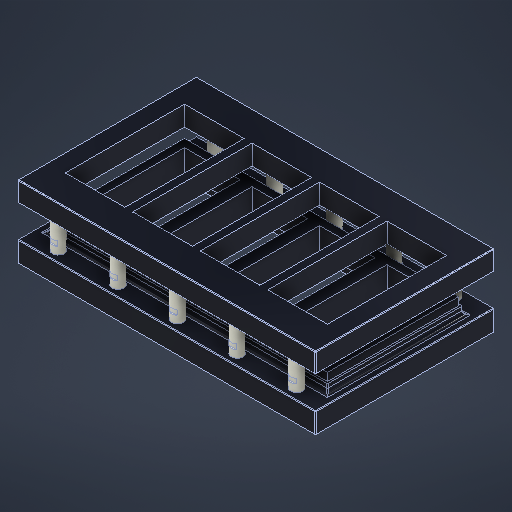
# Autodesk Inventor part: SACMI PH1500 30X60 DIE SET BASE
Saved by Autodesk Inventor 2025 (Build 290162000, 162)
## iProperties
Created: 2024-05-02
Part Number: SACMI PH1500 30X60 DIE SET BASE
Material: Generic
Document SubType Name: Modeling
Designer: zulet
Density: 1 g/cm^3
Appearance: Navy Blue
Author: zulet
Autodesk Inventor part; units mm, degrees
ref_plane "YZ Plane" through (0, 0, 0) normal (1, 0, 0) x (0, 1, 0)
ref_plane "XZ Plane" through (0, 0, 0) normal (0, 1, 0) x (-1, 0, 0)
ref_plane "XY Plane" through (0, 0, 0) normal (0, 0, 1) x (1, 0, 0)
sketch "Sketch1" plane through (0, 0, 0) normal (0, 1, 0) x (-1, 0, 0)
  line L0 (750, -450) -> (-750, -450)
  line L1 (-750, -450) -> (-750, 450)
  line L2 (-750, 450) -> (750, 450)
  line L3 (750, 450) -> (750, -450)
  line L4 (750, -450) -> (-750, 450) construction
  line L5 (-750, -450) -> (750, 450) construction
  point P0 (0, 0)
  dimension "d0" = 1500
  dimension "d1" = 900
  constraints: 12 end point, 2 midpoint, 2 parallel, 1 horizontal, 1 perpendicular
  measures "d0" distance of L1.end L2.end
  measures "d1" distance of L0.end L1.end
extrude "Extrusion1" add sketch "Sketch1" along normal blind 105
sketch "Sketch2" plane through (0, 105, 0) normal (0, 1, 0) x (1, 0, 0)
  line L0 (750, -450) -> (750, 450) construction
  line L1 (750, 0) -> (-750, 0) construction
  line L2 (-750, 450) -> (-750, -450) construction
  line L3 (660, -300) -> (360, -300) construction
  line L4 (360, -300) -> (360, 300) construction
  line L5 (360, 300) -> (660, 300) construction
  line L6 (660, 300) -> (660, -300) construction
  line L7 (660, -300) -> (360, 300) construction
  line L8 (360, -300) -> (660, 300) construction
  line L9 (370, -290) -> (650, -290)
  line L10 (650, -290) -> (650, 290)
  line L11 (650, 290) -> (370, 290)
  line L12 (370, 290) -> (370, -290)
  line L13 (30, -290) -> (310, -290)
  line L14 (30, 290) -> (30, -290)
  line L15 (20, -300) -> (20, 300) construction
  line L16 (20, -300) -> (320, 300) construction
  line L17 (320, -300) -> (20, -300) construction
  line L18 (320, -300) -> (20, 300) construction
  line L19 (320, 300) -> (320, -300) construction
  line L20 (310, 290) -> (30, 290)
  line L21 (20, 300) -> (320, 300) construction
  line L22 (310, -290) -> (310, 290)
  line L23 (-310, -290) -> (-30, -290)
  line L24 (-310, 290) -> (-310, -290)
  line L25 (-320, -300) -> (-320, 300) construction
  line L26 (-320, -300) -> (-20, 300) construction
  line L27 (-20, -300) -> (-320, -300) construction
  line L28 (-20, -300) -> (-320, 300) construction
  line L29 (-20, 300) -> (-20, -300) construction
  line L30 (-30, 290) -> (-310, 290)
  line L31 (-320, 300) -> (-20, 300) construction
  line L32 (-30, -290) -> (-30, 290)
  line L33 (-650, -290) -> (-370, -290)
  line L34 (-650, 290) -> (-650, -290)
  line L35 (-660, -300) -> (-660, 300) construction
  line L36 (-660, -300) -> (-360, 300) construction
  line L37 (-360, -300) -> (-660, -300) construction
  line L38 (-360, -300) -> (-660, 300) construction
  line L39 (-360, 300) -> (-360, -300) construction
  line L40 (-370, 290) -> (-650, 290)
  line L41 (-660, 300) -> (-360, 300) construction
  line L42 (-370, -290) -> (-370, 290)
  line L43 (-750, -450) -> (750, -450) projected
  line L44 (0, -450) -> (0, 450) construction
  line L45 (750, 450) -> (-750, 450) projected
  line L46 (-690, 330) -> (690, 330)
  line L47 (690, 330) -> (690, -330)
  line L48 (690, -330) -> (-690, -330)
  line L49 (-690, -330) -> (-690, 330)
  line L50 (-690, 330) -> (690, -330) construction
  line L51 (690, 330) -> (-690, -330) construction
  line L52 (-700, -340) -> (700, -340)
  line L53 (700, -340) -> (700, 340)
  line L54 (700, 340) -> (-700, 340)
  line L55 (-700, 340) -> (-700, -340)
  point P0 (0, 0)
  point P1 (510, 0)
  point P2 (170, 0)
  point P3 (-170, 0)
  point P4 (-510, 0)
  dimension "d4" = 300
  dimension "d5" = 600
  dimension "d6" = 10
  dimension "d9" = 340
  dimension "d14" = 30
  dimension "d15" = 30
  dimension "d16" = 10
  constraints: 104 end point, 8 midpoint, 8 parallel, 4 perpendicular, 3 horizontal, 1 point on line, 64 other
  measures "d4" distance of L4.end L5.end
  measures "d5" distance of L3.end L4.end
  measures "d6" distance between parallel lines of L3 L9
  measures "d9" distance of L9.start L13.start
  measures "d14" distance between parallel lines of L47 L6
  measures "d15" distance between parallel lines of L3 L48
  measures "d16" distance between parallel lines of L48 L52
extrude "Extrusion2" add sketch "Sketch2" along normal blind 40 contours L55 L54 L53 L52
extrude "Extrusion3" add sketch "Sketch2" along normal blind 80 contours L46 L47 L48 L49
extrude "Extrusion4" cut sketch "Sketch2" against normal through all contours L12 L11 L10 L9 | L14 L20 L22 L13 | L24 L30 L32 L23 | L34 L40 L42 L33
sketch "Sketch3" plane through (0, 0, 0) normal (0, -1, 0) x (1, 0, 0)
  line L0 (690, 330) -> (690, -330) projected
  line L1 (-690, 330) -> (690, 330)
  line L2 (690, 330) -> (690, -330)
  line L3 (690, -330) -> (-690, -330)
  line L4 (-690, -330) -> (-690, 330)
  line L5 (-690, 330) -> (690, -330) construction
  line L6 (690, 330) -> (-690, -330) construction
  point P0 (0, 0)
  constraints: 12 end point, 2 midpoint, 2 parallel, 1 horizontal, 1 perpendicular
extrude "Extrusion5" cut sketch "Sketch3" against normal blind 70
sketch "Sketch4" plane through (0, 105, 0) normal (0, 1, 0) x (1, 0, 0)
  circle A0 centre (600, -395) radius 30
  line L0 (-750, -450) -> (750, -450) projected
  line L1 (-750, 450) -> (-750, -450) projected
  line L2 (750, -450) -> (750, 450) projected
  line L3 (750, 450) -> (-750, 450) projected
  circle A1 centre (300, -395) radius 30
  circle A2 centre (0, -395) radius 30
  circle A3 centre (-300, -395) radius 30
  circle A4 centre (-600, -395) radius 30
  circle A5 centre (600, 395) radius 30
  circle A6 centre (300, 395) radius 30
  circle A7 centre (0, 395) radius 30
  circle A8 centre (-300, 395) radius 30
  circle A9 centre (-600, 395) radius 30
  line L4 (0, -395) -> (0, 395) construction
  point P0 (0, 0)
  point P1 (0, 0)
  dimension "d25" = 60
  dimension "d28" = 300
  dimension "d31" = 790
  constraints: 10 centre point, 2 end point, 2 vertical, 1 coincident, 1 horizontal, 1 midpoint, 18 other
  measures "d25" diameter of A0
  measures "d28" distance of A0.centre A1.centre
  measures "d31" distance of A0.centre A5.centre
extrude "Extrusion6" add sketch "Sketch4" along normal blind 160 contours A0 | A1 | A2 | A3 | A4 | A5 | A6 | A7 | A8 | A9
sketch "Sketch5" plane through (600, 265, 395) normal (0, 1, 0) x (1, 0, 0)
  line L0 (-1350, 845) -> (150, 845)
  line L1 (150, 845) -> (150, -55)
  line L2 (150, -55) -> (-1350, -55)
  line L3 (-1350, -55) -> (-1350, 845)
  line L4 (-1350, 845) -> (150, -55) construction
  line L5 (150, 845) -> (-1350, -55) construction
  line L6 (-290, 105) -> (-570, 105) construction
  line L7 (-290, 685) -> (-290, 105) construction
  line L8 (-570, 105) -> (-570, 685) construction
  line L9 (-570, 685) -> (-290, 685) construction
  line L10 (-230, 105) -> (-230, 685) construction
  line L11 (50, 105) -> (-230, 105) construction
  line L12 (50, 685) -> (50, 105) construction
  line L13 (-230, 685) -> (50, 685) construction
  line L14 (-630, 685) -> (-630, 105) construction
  line L15 (-630, 105) -> (-910, 105) construction
  line L16 (-910, 105) -> (-910, 685) construction
  line L17 (-910, 685) -> (-630, 685) construction
  line L18 (-970, 685) -> (-970, 105) construction
  line L19 (-970, 105) -> (-1250, 105) construction
  line L20 (-1250, 105) -> (-1250, 685) construction
  line L21 (-1250, 685) -> (-970, 685) construction
  line L22 (-240, 95) -> (-240, 695)
  line L23 (-240, 695) -> (60, 695)
  line L24 (60, 695) -> (60, 95)
  line L25 (60, 95) -> (-240, 95)
  line L26 (-620, 95) -> (-620, 695)
  line L27 (-620, 695) -> (-920, 695)
  line L28 (-920, 695) -> (-920, 95)
  line L29 (-920, 95) -> (-620, 95)
  line L30 (-960, 95) -> (-960, 695)
  line L31 (-960, 695) -> (-1260, 695)
  line L32 (-1260, 695) -> (-1260, 95)
  line L33 (-1260, 95) -> (-960, 95)
  line L34 (-280, 95) -> (-580, 95)
  line L35 (-580, 95) -> (-580, 695)
  line L36 (-580, 695) -> (-280, 695)
  line L37 (-280, 695) -> (-280, 95)
  point P0 (-600, 395)
  dimension "d36" = 1500
  dimension "d37" = 900
  dimension "d38" = 10
  dimension "d40" = 10
  dimension "d41" = 10
  dimension "d42" = 10
  constraints: 44 end point, 2 midpoint, 2 parallel, 1 horizontal, 1 perpendicular, 12 other
  measures "d36" distance of L1.end L2.end
  measures "d37" distance of L0.end L1.end
  measures "d38" distance between parallel lines of L11 L25
  measures "d40" distance between parallel lines of L14 L26
  measures "d41" distance between parallel lines of L18 L30
  measures "d42" distance between parallel lines of L7 L37
extrude "Extrusion7" add sketch "Sketch5" along normal blind 100
fillet "Fillet1" radius 20 4 edges at (700, 105, 0) (0, 105, -340) (0, 105, 340) (-700, 105, 0)
sketch "Sketch6" plane through (750, 0, 450) normal (1, 0, 0) x (0, 0, -1)
  line L0 (32.5, 142.5) -> (17.5, 142.5)
  line L1 (17.5, 142.5) -> (17.5, 167.5)
  line L2 (17.5, 167.5) -> (32.5, 167.5)
  line L3 (32.5, 167.5) -> (32.5, 142.5)
  line L4 (32.5, 142.5) -> (17.5, 167.5) construction
  line L5 (17.5, 142.5) -> (32.5, 167.5) construction
  line L6 (25, 105) -> (25, 265) projected
  line L7 (0, 105) -> (900, 105) projected
  line L8 (450, 0) -> (450, 105) construction
  line L9 (867.5, 142.5) -> (882.5, 142.5)
  line L10 (882.5, 142.5) -> (882.5, 167.5)
  line L11 (882.5, 167.5) -> (867.5, 167.5)
  line L12 (867.5, 167.5) -> (867.5, 142.5)
  line L13 (875, 105) -> (875, 265)
  point P0 (25, 155)
  dimension "d46" = 15
  dimension "d47" = 25
  dimension "d48" = 50
  constraints: 24 end point, 6 symmetric about line, 3 midpoint, 2 parallel, 1 horizontal, 1 perpendicular, 1 point on line
  measures "d46" distance of L1.end L2.end
  measures "d47" distance of L0.end L1.end
  measures "d48" distance from line of L7 point (25, 155)
extrude "Extrusion8" cut sketch "Sketch6" against normal through all
fillet "Fillet2" radius 3 12 edges at (0, 365, 450) (750, 315, 450) (0, 265, 450) (-750, 315, 450) (-750, 365, 0) (-750, 315, -450) (-750, 265, 0) (0, 365, -450) (750, 365, 0) (750, 265, 0) (750, 315, -450) (0, 265, -450)
fillet "Fillet3" radius 3 12 edges at (750, 52.5, -450) (0, 105, -450) (0, 0, -450) (-750, 52.5, -450) (-750, 105, 0) (750, 105, 0) (750, 52.5, 450) (750, 0, 0) (0, 105, 450) (0, 0, 450) (-750, 0, 0) (-750, 52.5, 450)
fillet "Fillet4" radius 5 8 edges at (705.8579, 110.8579, -345.8579) (700, 135, -340) (705.8579, 110.8579, 345.8579) (700, 135, 340) (-705.8579, 110.8579, -345.8579) (-700, 135, -340) (-705.8579, 110.8579, 345.8579) (-700, 135, 340)
sketch "Sketch7" plane through (747, 3, -450) normal (0, 0, -1) x (-1, 0, 0)
  circle A0 centre (267, 49.5) radius 20
  circle A1 centre (387, 49.5) radius 20
  line L0 (267, 49.5) -> (387, 49.5) construction
  line L1 (1494, 99) -> (0, 99) construction
  line L2 (327, 99) -> (327, 0) construction
  line L3 (0, 0) -> (1494, 0) construction
  line L4 (747, 0) -> (747, 99) construction
  circle A2 centre (1227, 49.5) radius 20
  circle A3 centre (1107, 49.5) radius 20
  point P0 (747, -3)
  point P1 (327, 49.5)
  dimension "d54" = 40
  dimension "d55" = 40
  dimension "d56" = 420
  dimension "d57" = 120
  constraints: 6 end point, 4 centre point, 4 midpoint, 2 point on line, 2 symmetric about line, 1 horizontal, 1 vertical, 2 other
  measures "d54" diameter of A0
  measures "d55" diameter of A1
  measures "d56" horizontal distance of L4.start point (327, 49.5)
  measures "d57" distance of L0.start L0.end
extrude "Extrusion9" cut sketch "Sketch7" against normal blind 20
body "Solid1"
